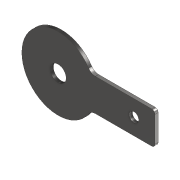
# Autodesk Inventor part: stelscharnier onderkant
Saved by Autodesk Inventor 2020.3 (Build 243373000, 373)
## iProperties
Created: 2020-09-15
Part Number: stelscharnier onderkant
Material: Stainless Steel
Document SubType Name: Modeling
Designer: Svend
Density: 8 g/cm^3
Appearance: Semi-Polished
Author: Svend
Autodesk Inventor part; units mm, degrees
ref_plane "YZ Plane" through (0, 0, 0) normal (1, 0, 0) x (0, 1, 0)
ref_plane "XZ Plane" through (0, 0, 0) normal (0, 1, 0) x (-1, 0, 0)
ref_plane "XY Plane" through (0, 0, 0) normal (0, 0, 1) x (1, 0, 0)
sketch "Sketch1" plane through (0, 0, 0) normal (0, 0, 1) x (1, 0, 0)
  circle A0 centre (0, 0) radius 22.5
  line L0 (162.5, 0) -> (-22.5, 0) construction
  circle A1 centre (0, 0) radius 5
  line L1 (60, 10) -> (20.1556, 10)
  line L2 (20.1556, 10) -> (20.1556, -10)
  line L3 (20.1556, -10) -> (60, -10)
  line L4 (60, -10) -> (60, 10)
  circle A2 centre (47, 0) radius 3
  point P0 (6.3, 21.6)
  point P1 (60, 0)
  dimension "d0" = 45
  dimension "d3" = 10
  dimension "d7" = 20
  dimension "d8" = 60
  dimension "d9" = 6
  dimension "d10" = 13
  constraints: 10 end point, 3 centre point, 3 point on circle, 2 coincident, 2 horizontal, 2 parallel, 2 point on line, 1 horizontal alignment, 1 midpoint, 1 perpendicular
  measures "d0" diameter of A0
  measures "d3" diameter of A1
  measures "d7" distance between parallel lines of L3 L1
  measures "d8" distance from line of A1.centre L4
  measures "d9" diameter of A2
  measures "d10" distance from line of L4 A2.centre
extrude "Extrusion1" add sketch "Sketch1" along normal mid plane 2
fillet "Fillet1" radius 5 2 edges at (20.1556, 10, 0) (20.1556, -10, 0)
fillet "Fillet2" radius 2 2 edges at (60, -10, 0) (60, 10, 0)
body "Solid1"
